Autodesk Fusion 360 part; units mm, degrees
note: some values were not read from the file. Set by a fixed rule: which sketch regions a step uses.
(part 6 of 59)
  spline S28 degree 5 poles (-28.1181, -0.5527) (-28.1154, -0.5525) (-28.11, -0.5521) (-28.1019, -0.5515) (-28.0911, -0.5506) (-28.0777, -0.5495) (-28.0644, -0.5484) (-28.051, -0.5473) (-28.0377, -0.5462) (-28.0244, -0.5451) (-28.0112, -0.5439) (-27.9979, -0.5427) (-27.9848, -0.5415) (-27.9716, -0.5404) (-27.9585, -0.5391) (-27.9454, -0.5379) (-27.9323, -0.5367) (-27.9193, -0.5354) (-27.9063, -0.5342) (-27.8934, -0.5329) (-27.8805, -0.5316) (-27.8676, -0.5303) (-27.8547, -0.529) (-27.8419, -0.5276) (-27.8291, -0.5263) (-27.8164, -0.5249) (-27.8037, -0.5236) (-27.791, -0.5222) (-27.7784, -0.5208) (-27.7658, -0.5194) (-27.7532, -0.518) (-27.7406, -0.5165) (-27.7281, -0.5151) (-27.7157, -0.5136) (-27.7032, -0.5122) (-27.6908, -0.5107) (-27.6785, -0.5092) (-27.6661, -0.5077) (-27.6539, -0.5062) (-27.6416, -0.5047) (-27.6294, -0.5031) (-27.6172, -0.5016) (-27.605, -0.5) (-27.5929, -0.4984) (-27.5809, -0.4968) (-27.5688, -0.4952) (-27.5568, -0.4936) (-27.5449, -0.492) (-27.5329, -0.4904) (-27.521, -0.4887) (-27.5092, -0.4871) (-27.4974, -0.4854) (-27.4856, -0.4838) (-27.4738, -0.4821) (-27.4621, -0.4804) (-27.4505, -0.4787) (-27.4388, -0.477) (-27.4273, -0.4752) (-27.4157, -0.4735) (-27.4042, -0.4718) (-27.3927, -0.47) (-27.3813, -0.4682) (-27.3699, -0.4665) (-27.3585, -0.4647) (-27.3472, -0.4629) (-27.3359, -0.4611) (-27.3247, -0.4593) (-27.3135, -0.4574) (-27.3023, -0.4556) (-27.2912, -0.4538) (-27.2801, -0.4519) (-27.2691, -0.4501) (-27.2581, -0.4482) (-27.2471, -0.4463) (-27.2362, -0.4445) (-27.2253, -0.4426) (-27.2145, -0.4407) (-27.2037, -0.4388) (-27.1929, -0.4368) (-27.1822, -0.4349) (-27.1715, -0.433) (-27.1609, -0.4311) (-27.1503, -0.4291) (-27.1397, -0.4272) (-27.1292, -0.4252) (-27.1188, -0.4232) (-27.1083, -0.4213) (-27.0979, -0.4193) (-27.0876, -0.4173) (-27.0773, -0.4153) (-27.0671, -0.4133) (-27.0568, -0.4113) (-27.0467, -0.4093) (-27.0365, -0.4072) (-27.0265, -0.4052) (-27.0164, -0.4032) (-27.0064, -0.4011) (-26.9965, -0.3991) (-26.9866, -0.3971) (-26.9767, -0.395) (-26.9669, -0.3929) (-26.9571, -0.3909) (-26.9474, -0.3888) (-26.9377, -0.3867) (-26.9281, -0.3847) (-26.9185, -0.3826) (-26.9089, -0.3805) (-26.8994, -0.3784) (-26.89, -0.3763) (-26.8806, -0.3742) (-26.8712, -0.3721) (-26.8619, -0.37) (-26.8526, -0.3679) (-26.8434, -0.3658) (-26.8342, -0.3636) (-26.8251, -0.3615) (-26.816, -0.3594) (-26.8069, -0.3573) (-26.798, -0.3551) (-26.789, -0.353) (-26.7801, -0.3509) (-26.7713, -0.3487) (-26.7625, -0.3466) (-26.7537, -0.3445) (-26.7451, -0.3423) (-26.7364, -0.3402) (-26.7278, -0.338) (-26.7193, -0.3359) (-26.7108, -0.3337) (-26.7023, -0.3316) (-26.6939, -0.3294) (-26.6856, -0.3273) (-26.6773, -0.3251) (-26.669, -0.323) (-26.6608, -0.3208) (-26.6527, -0.3187) (-26.6446, -0.3166) (-26.6365, -0.3144) (-26.6286, -0.3123) (-26.6206, -0.3101) (-26.6127, -0.308) (-26.6049, -0.3058) (-26.5971, -0.3037) (-26.5894, -0.3016) (-26.5817, -0.2994) (-26.5741, -0.2973) (-26.5665, -0.2952) (-26.559, -0.293) (-26.5516, -0.2909) (-26.5442, -0.2888) (-26.5368, -0.2867) (-26.5296, -0.2845) (-26.5223, -0.2824) (-26.5151, -0.2803) (-26.508, -0.2782) (-26.5009, -0.2761) (-26.4939, -0.274) (-26.487, -0.272) (-26.4801, -0.2699) (-26.4733, -0.2678) (-26.4665, -0.2657) (-26.4598, -0.2637) (-26.4531, -0.2616) (-26.4465, -0.2596) (-26.4399, -0.2575) (-26.4335, -0.2555) (-26.427, -0.2534) (-26.4207, -0.2514) (-26.4144, -0.2494) (-26.4081, -0.2474) (-26.4019, -0.2454) (-26.3958, -0.2434) (-26.3897, -0.2414) (-26.3837, -0.2395) (-26.3778, -0.2375) (-26.3719, -0.2356) (-26.3661, -0.2336) (-26.3604, -0.2317) (-26.3547, -0.2298) (-26.3491, -0.2279) (-26.3435, -0.226) (-26.338, -0.2241) (-26.3326, -0.2222) (-26.3273, -0.2204) (-26.322, -0.2185) (-26.3167, -0.2167) (-26.3116, -0.2149) (-26.3065, -0.2131) (-26.3015, -0.2113) (-26.2965, -0.2095) (-26.2916, -0.2077) (-26.2868, -0.206) (-26.282, -0.2043) (-26.2774, -0.2026) (-26.2728, -0.2009) (-26.2682, -0.1992) (-26.2638, -0.1975) (-26.2594, -0.1959) (-26.255, -0.1943) (-26.2508, -0.1927) (-26.2466, -0.1911) (-26.2425, -0.1895) (-26.2385, -0.188) (-26.2345, -0.1864) (-26.2307, -0.1849) (-26.2269, -0.1834) (-26.2231, -0.182) (-26.2195, -0.1806) (-26.2159, -0.1791) (-26.2124, -0.1778) (-26.209, -0.1764) (-26.2057, -0.175) (-26.2024, -0.1737) (-26.1993, -0.1724) (-26.1962, -0.1712) (-26.1932, -0.1699) (-26.1903, -0.1687) (-26.1874, -0.1676) (-26.1847, -0.1664) (-26.182, -0.1653) (-26.1794, -0.1642) (-26.1769, -0.1631) (-26.1745, -0.1621) (-26.1722, -0.1611) (-26.17, -0.1602) (-26.1678, -0.1592) (-26.1658, -0.1583) (-26.1638, -0.1575) (-26.1619, -0.1567) (-26.1602, -0.1559) (-26.1585, -0.1551) (-26.1569, -0.1544) (-26.1554, -0.1538) (-26.154, -0.1531) (-26.1527, -0.1526) (-26.1515, -0.152) (-26.1504, -0.1515) (-26.1495, -0.151) (-26.1486, -0.1506) (-26.1478, -0.1503) (-26.1471, -0.15) (-26.1467, -0.1497) (-26.1464, -0.1496) (-26.1462, -0.1495) (-26.1461, -0.1495) knots -1 -1 -1 -1 -1 -1 -0.99583333 -0.99166667 -0.9875 -0.98333333 -0.97916667 -0.975 -0.97083333 -0.96666667 -0.9625 -0.95833333 -0.95416667 -0.95 -0.94583333 -0.94166667 -0.9375 -0.93333333 -0.92916667 -0.925 -0.92083333 -0.91666667 -0.9125 -0.90833333 -0.90416667 -0.9 -0.89583333 -0.89166667 -0.8875 -0.88333333 -0.87916667 -0.875 -0.87083333 -0.86666667 -0.8625 -0.85833333 -0.85416667 -0.85 -0.84583333 -0.84166667 -0.8375 -0.83333333 -0.82916667 -0.825 -0.82083333 -0.81666667 -0.8125 -0.80833333 -0.80416667 -0.8 -0.79583333 -0.79166667 -0.7875 -0.78333333 -0.77916667 -0.775 -0.77083333 -0.76666667 -0.7625 -0.75833333 -0.75416667 -0.75 -0.74583333 -0.74166667 -0.7375 -0.73333333 -0.72916667 -0.725 -0.72083333 -0.71666667 -0.7125 -0.70833333 -0.70416667 -0.7 -0.69583333 -0.69166667 -0.6875 -0.68333333 -0.67916667 -0.675 -0.67083333 -0.66666667 -0.6625 -0.65833333 -0.65416667 -0.65 -0.64583333 -0.64166667 -0.6375 -0.63333333 -0.62916667 -0.625 -0.62083333 -0.61666667 -0.6125 -0.60833333 -0.60416667 -0.6 -0.59583333 -0.59166667 -0.5875 -0.58333333 -0.57916667 -0.575 -0.57083333 -0.56666667 -0.5625 -0.55833333 -0.55416667 -0.55 -0.54583333 -0.54166667 -0.5375 -0.53333333 -0.52916667 -0.525 -0.52083333 -0.51666667 -0.5125 -0.50833333 -0.50416667 -0.5 -0.49583333 -0.49166667 -0.4875 -0.48333333 -0.47916667 -0.475 -0.47083333 -0.46666667 -0.4625 -0.45833333 -0.45416667 -0.45 -0.44583333 -0.44166667 -0.4375 -0.43333333 -0.42916667 -0.425 -0.42083333 -0.41666667 -0.4125 -0.40833333 -0.40416667 -0.4 -0.39583333 -0.39166667 -0.3875 -0.38333333 -0.37916667 -0.375 -0.37083333 -0.36666667 -0.3625 -0.35833333 -0.35416667 -0.35 -0.34583333 -0.34166667 -0.3375 -0.33333333 -0.32916667 -0.325 -0.32083333 -0.31666667 -0.3125 -0.30833333 -0.30416667 -0.3 -0.29583333 -0.29166667 -0.2875 -0.28333333 -0.27916667 -0.275 -0.27083333 -0.26666667 -0.2625 -0.25833333 -0.25416667 -0.25 -0.24583333 -0.24166667 -0.2375 -0.23333333 -0.22916667 -0.225 -0.22083333 -0.21666667 -0.2125 -0.20833333 -0.20416667 -0.2 -0.19583333 -0.19166667 -0.1875 -0.18333333 -0.17916667 -0.175 -0.17083333 -0.16666667 -0.1625 -0.15833333 -0.15416667 -0.15 -0.14583333 -0.14166667 -0.1375 -0.13333333 -0.12916667 -0.125 -0.12083333 -0.11666667 -0.1125 -0.10833333 -0.10416667 -0.1 -0.09583333 -0.09166667 -0.0875 -0.08333333 -0.07916667 -0.075 -0.07083333 -0.06666667 -0.0625 -0.05833333 -0.05416667 -0.05 -0.04583333 -0.04166667 -0.0375 -0.03333333 -0.02916667 -0.025 -0.02083333 -0.01666667 -0.0125 -0.00833333 -0.00416667 0 0 0 0 0 0
  spline S29 degree 5 poles (-27.3251, 22.3472) (-27.3252, 22.3472) (-27.3254, 22.3473) (-27.3257, 22.3474) (-27.3262, 22.3475) (-27.3269, 22.3478) (-27.3277, 22.3481) (-27.3286, 22.3484) (-27.3296, 22.3487) (-27.3308, 22.3491) (-27.332, 22.3495) (-27.3334, 22.35) (-27.3348, 22.3505) (-27.3364, 22.351) (-27.338, 22.3515) (-27.3398, 22.3521) (-27.3416, 22.3527) (-27.3435, 22.3533) (-27.3456, 22.3539) (-27.3477, 22.3546) (-27.3499, 22.3553) (-27.3523, 22.356) (-27.3547, 22.3568) (-27.3572, 22.3575) (-27.3598, 22.3583) (-27.3625, 22.3591) (-27.3652, 22.36) (-27.3681, 22.3608) (-27.371, 22.3617) (-27.3741, 22.3626) (-27.3772, 22.3635) (-27.3804, 22.3645) (-27.3837, 22.3654) (-27.387, 22.3664) (-27.3905, 22.3674) (-27.394, 22.3684) (-27.3976, 22.3694) (-27.4013, 22.3704) (-27.4051, 22.3715) (-27.409, 22.3725) (-27.4129, 22.3736) (-27.4169, 22.3747) (-27.421, 22.3758) (-27.4252, 22.3769) (-27.4294, 22.378) (-27.4337, 22.3792) (-27.4381, 22.3803) (-27.4426, 22.3815) (-27.4471, 22.3827) (-27.4517, 22.3838) (-27.4564, 22.385) (-27.4612, 22.3862) (-27.466, 22.3874) (-27.4709, 22.3887) (-27.4759, 22.3899) (-27.481, 22.3911) (-27.4861, 22.3924) (-27.4912, 22.3936) (-27.4965, 22.3949) (-27.5018, 22.3962) (-27.5072, 22.3974) (-27.5127, 22.3987) (-27.5182, 22.4) (-27.5238, 22.4013) (-27.5294, 22.4026) (-27.5352, 22.4039) (-27.5409, 22.4052) (-27.5468, 22.4065) (-27.5527, 22.4079) (-27.5587, 22.4092) (-27.5647, 22.4105) (-27.5709, 22.4118) (-27.577, 22.4132) (-27.5833, 22.4145) (-27.5896, 22.4158) (-27.5959, 22.4172) (-27.6023, 22.4185) (-27.6088, 22.4199) (-27.6154, 22.4212) (-27.622, 22.4225) (-27.6286, 22.4239) (-27.6353, 22.4252) (-27.6421, 22.4266) (-27.649, 22.4279) (-27.6559, 22.4293) (-27.6628, 22.4306) (-27.6698, 22.432) (-27.6769, 22.4333) (-27.6841, 22.4347) (-27.6912, 22.436) (-27.6985, 22.4374) (-27.7058, 22.4387) (-27.7132, 22.4401) (-27.7206, 22.4414) (-27.728, 22.4428) (-27.7356, 22.4441) (-27.7431, 22.4454) (-27.7508, 22.4468) (-27.7585, 22.4481) (-27.7662, 22.4494) (-27.774, 22.4508) (-27.7819, 22.4521) (-27.7898, 22.4534) (-27.7977, 22.4547) (-27.8057, 22.456) (-27.8138, 22.4573) (-27.8219, 22.4586) (-27.8301, 22.4599) (-27.8383, 22.4612) (-27.8466, 22.4625) (-27.8549, 22.4638) (-27.8633, 22.4651) (-27.8717, 22.4664) (-27.8802, 22.4676) (-27.8887, 22.4689) (-27.8973, 22.4701) (-27.9059, 22.4714) (-27.9146, 22.4726) (-27.9233, 22.4739) (-27.9321, 22.4751) (-27.9409, 22.4763) (-27.9498, 22.4776) (-27.9587, 22.4788) (-27.9677, 22.48) (-27.9767, 22.4812) (-27.9858, 22.4824) (-27.9949, 22.4836) (-28.004, 22.4847) (-28.0133, 22.4859) (-28.0225, 22.4871) (-28.0318, 22.4882) (-28.0412, 22.4894) (-28.0506, 22.4905) (-28.06, 22.4916) (-28.0695, 22.4928) (-28.079, 22.4939) (-28.0886, 22.495) (-28.0982, 22.4961) (-28.1079, 22.4972) (-28.1176, 22.4983) (-28.1274, 22.4993) (-28.1372, 22.5004) (-28.147, 22.5014) (-28.1569, 22.5025) (-28.1668, 22.5035) (-28.1768, 22.5045) (-28.1868, 22.5055) (-28.1969, 22.5065) (-28.207, 22.5075) (-28.2172, 22.5085) (-28.2274, 22.5095) (-28.2376, 22.5104) (-28.2479, 22.5114) (-28.2582, 22.5123) (-28.2686, 22.5133) (-28.279, 22.5142) (-28.2894, 22.5151) (-28.2999, 22.516) (-28.3105, 22.5169) (-28.321, 22.5177) (-28.3317, 22.5186) (-28.3423, 22.5195) (-28.353, 22.5203) (-28.3638, 22.5211) (-28.3745, 22.5219) (-28.3854, 22.5227) (-28.3962, 22.5235) (-28.4071, 22.5243) (-28.4181, 22.5251) (-28.429, 22.5258) (-28.44, 22.5266) (-28.4511, 22.5273) (-28.4622, 22.528) (-28.4733, 22.5287) (-28.4845, 22.5294) (-28.4957, 22.5301) (-28.507, 22.5308) (-28.5183, 22.5314) (-28.5296, 22.5321) (-28.541, 22.5327) (-28.5524, 22.5333) (-28.5638, 22.5339) (-28.5753, 22.5345) (-28.5868, 22.5351) (-28.5984, 22.5356) (-28.61, 22.5362) (-28.6216, 22.5367) (-28.6333, 22.5372) (-28.645, 22.5377) (-28.6567, 22.5382) (-28.6685, 22.5387) (-28.6803, 22.5392) (-28.6922, 22.5396) (-28.7041, 22.54) (-28.716, 22.5405) (-28.728, 22.5409) (-28.74, 22.5412) (-28.752, 22.5416) (-28.7641, 22.542) (-28.7762, 22.5423) (-28.7883, 22.5427) (-28.8005, 22.543) (-28.8127, 22.5433) (-28.8249, 22.5436) (-28.8372, 22.5438) (-28.8495, 22.5441) (-28.8619, 22.5443) (-28.8743, 22.5445) (-28.8867, 22.5448) (-28.8991, 22.5449) (-28.9116, 22.5451) (-28.9241, 22.5453) (-28.9367, 22.5454) (-28.9493, 22.5456) (-28.9619, 22.5457) (-28.9745, 22.5458) (-28.9872, 22.5458) (-29, 22.5459) (-29.0127, 22.546) (-29.0255, 22.546) (-29.0383, 22.546) (-29.0512, 22.546) (-29.0641, 22.546) (-29.077, 22.546) (-29.0899, 22.5459) (-29.1029, 22.5458) (-29.1159, 22.5458) (-29.129, 22.5457) (-29.142, 22.5455) (-29.1551, 22.5454) (-29.1683, 22.5453) (-29.1815, 22.5451) (-29.1947, 22.5449) (-29.2079, 22.5447) (-29.2212, 22.5445) (-29.2345, 22.5442) (-29.2478, 22.544) (-29.2612, 22.5437) (-29.2745, 22.5434) (-29.288, 22.5431) (-29.3014, 22.5428) (-29.3122, 22.5425) (-29.3203, 22.5423) (-29.3257, 22.5422) (-29.3284, 22.5421) knots 0 0 0 0 0 0 0.00416667 0.00833333 0.0125 0.01666667 0.02083333 0.025 0.02916667 0.03333333 0.0375 0.04166667 0.04583333 0.05 0.05416667 0.05833333 0.0625 0.06666667 0.07083333 0.075 0.07916667 0.08333333 0.0875 0.09166667 0.09583333 0.1 0.10416667 0.10833333 0.1125 0.11666667 0.12083333 0.125 0.12916667 0.13333333 0.1375 0.14166667 0.14583333 0.15 0.15416667 0.15833333 0.1625 0.16666667 0.17083333 0.175 0.17916667 0.18333333 0.1875 0.19166667 0.19583333 0.2 0.20416667 0.20833333 0.2125 0.21666667 0.22083333 0.225 0.22916667 0.23333333 0.2375 0.24166667 0.24583333 0.25 0.25416667 0.25833333 0.2625 0.26666667 0.27083333 0.275 0.27916667 0.28333333 0.2875 0.29166667 0.29583333 0.3 0.30416667 0.30833333 0.3125 0.31666667 0.32083333 0.325 0.32916667 0.33333333 0.3375 0.34166667 0.34583333 0.35 0.35416667 0.35833333 0.3625 0.36666667 0.37083333 0.375 0.37916667 0.38333333 0.3875 0.39166667 0.39583333 0.4 0.40416667 0.40833333 0.4125 0.41666667 0.42083333 0.425 0.42916667 0.43333333 0.4375 0.44166667 0.44583333 0.45 0.45416667 0.45833333 0.4625 0.46666667 0.47083333 0.475 0.47916667 0.48333333 0.4875 0.49166667 0.49583333 0.5 0.50416667 0.50833333 0.5125 0.51666667 0.52083333 0.525 0.52916667 0.53333333 0.5375 0.54166667 0.54583333 0.55 0.55416667 0.55833333 0.5625 0.56666667 0.57083333 0.575 0.57916667 0.58333333 0.5875 0.59166667 0.59583333 0.6 0.60416667 0.60833333 0.6125 0.61666667 0.62083333 0.625 0.62916667 0.63333333 0.6375 0.64166667 0.64583333 0.65 0.65416667 0.65833333 0.6625 0.66666667 0.67083333 0.675 0.67916667 0.68333333 0.6875 0.69166667 0.69583333 0.7 0.70416667 0.70833333 0.7125 0.71666667 0.72083333 0.725 0.72916667 0.73333333 0.7375 0.74166667 0.74583333 0.75 0.75416667 0.75833333 0.7625 0.76666667 0.77083333 0.775 0.77916667 0.78333333 0.7875 0.79166667 0.79583333 0.8 0.80416667 0.80833333 0.8125 0.81666667 0.82083333 0.825 0.82916667 0.83333333 0.8375 0.84166667 0.84583333 0.85 0.85416667 0.85833333 0.8625 0.86666667 0.87083333 0.875 0.87916667 0.88333333 0.8875 0.89166667 0.89583333 0.9 0.90416667 0.90833333 0.9125 0.91666667 0.92083333 0.925 0.92916667 0.93333333 0.9375 0.94166667 0.94583333 0.95 0.95416667 0.95833333 0.9625 0.96666667 0.97083333 0.975 0.97916667 0.98333333 0.9875 0.99166667 0.99583333 1 1 1 1 1 1
  spline S30 degree 5 poles (-25.6019, -1.2175) (-25.602, -1.2175) (-25.6022, -1.2176) (-25.6025, -1.2178) (-25.6029, -1.218) (-25.6036, -1.2184) (-25.6043, -1.2188) (-25.6052, -1.2193) (-25.6061, -1.2198) (-25.6072, -1.2204) (-25.6083, -1.221) (-25.6096, -1.2217) (-25.6109, -1.2225) (-25.6123, -1.2233) (-25.6138, -1.2242) (-25.6154, -1.2251) (-25.6171, -1.2261) (-25.6188, -1.2271) (-25.6207, -1.2282) (-25.6226, -1.2293) (-25.6246, -1.2305) (-25.6267, -1.2317) (-25.6289, -1.233) (-25.6311, -1.2344) (-25.6334, -1.2358) (-25.6358, -1.2372) (-25.6383, -1.2387) (-25.6409, -1.2403) (-25.6435, -1.2419) (-25.6462, -1.2435) (-25.6489, -1.2452) (-25.6518, -1.247) (-25.6547, -1.2488) (-25.6577, -1.2506) (-25.6607, -1.2526) (-25.6638, -1.2545) (-25.667, -1.2565) (-25.6702, -1.2586) (-25.6735, -1.2607) (-25.6769, -1.2628) (-25.6803, -1.265) (-25.6838, -1.2673) (-25.6874, -1.2696) (-25.691, -1.2719) (-25.6947, -1.2743) (-25.6984, -1.2768) (-25.7022, -1.2793) (-25.706, -1.2818) (-25.71, -1.2844) (-25.7139, -1.287) (-25.718, -1.2897) (-25.722, -1.2925) (-25.7262, -1.2952) (-25.7304, -1.2981) (-25.7346, -1.3009) (-25.7389, -1.3039) (-25.7432, -1.3068) (-25.7476, -1.3098) (-25.7521, -1.3129) (-25.7566, -1.316) (-25.7612, -1.3192) (-25.7658, -1.3224) (-25.7704, -1.3256) (-25.7751, -1.3289) (-25.7799, -1.3322) (-25.7847, -1.3356) (-25.7895, -1.339) (-25.7944, -1.3425) (-25.7993, -1.346) (-25.8043, -1.3496) (-25.8093, -1.3532) (-25.8144, -1.3568) (-25.8195, -1.3605) (-25.8247, -1.3643) (-25.8299, -1.3681) (-25.8352, -1.3719) (-25.8405, -1.3758) (-25.8458, -1.3797) (-25.8512, -1.3836) (-25.8566, -1.3876) (-25.8621, -1.3917) (-25.8676, -1.3958) (-25.8731, -1.3999) (-25.8787, -1.4041) (-25.8843, -1.4083) (-25.89, -1.4126) (-25.8957, -1.4169) (-25.9014, -1.4213) (-25.9072, -1.4257) (-25.913, -1.4301) (-25.9188, -1.4346) (-25.9247, -1.4391) (-25.9306, -1.4437) (-25.9366, -1.4483) (-25.9426, -1.4529) (-25.9486, -1.4576) (-25.9547, -1.4624) (-25.9608, -1.4672) (-25.9669, -1.472) (-25.9731, -1.4769) (-25.9793, -1.4818) (-25.9855, -1.4867) (-25.9918, -1.4917) (-25.9981, -1.4967) (-26.0044, -1.5018) (-26.0108, -1.5069) (-26.0172, -1.5121) (-26.0236, -1.5173) (-26.0301, -1.5225) (-26.0366, -1.5278) (-26.0431, -1.5332) (-26.0497, -1.5385) (-26.0563, -1.5439) (-26.0629, -1.5494) (-26.0695, -1.5549) (-26.0762, -1.5604) (-26.0829, -1.566) (-26.0896, -1.5716) (-26.0964, -1.5772) (-26.1032, -1.5829) (-26.11, -1.5887) (-26.1168, -1.5945) (-26.1237, -1.6003) (-26.1306, -1.6061) (-26.1375, -1.612) (-26.1445, -1.618) (-26.1515, -1.6239) (-26.1585, -1.63) (-26.1655, -1.636) (-26.1726, -1.6421) (-26.1796, -1.6483) (-26.1868, -1.6544) (-26.1939, -1.6607) (-26.201, -1.6669) (-26.2082, -1.6732) (-26.2154, -1.6796) (-26.2227, -1.6859) (-26.2299, -1.6924) (-26.2372, -1.6988) (-26.2445, -1.7053) (-26.2518, -1.7119) (-26.2592, -1.7184) (-26.2665, -1.725) (-26.2739, -1.7317) (-26.2813, -1.7384) (-26.2888, -1.7451) (-26.2962, -1.7519) (-26.3037, -1.7587) (-26.3112, -1.7656) (-26.3188, -1.7724) (-26.3263, -1.7794) (-26.3339, -1.7863) (-26.3414, -1.7933) (-26.3491, -1.8004) (-26.3567, -1.8075) (-26.3643, -1.8146) (-26.372, -1.8217) (-26.3797, -1.8289) (-26.3874, -1.8362) (-26.3951, -1.8435) (-26.4029, -1.8508) (-26.4106, -1.8581) (-26.4184, -1.8655) (-26.4262, -1.8729) (-26.434, -1.8804) (-26.4419, -1.8879) (-26.4497, -1.8954) (-26.4576, -1.903) (-26.4655, -1.9106) (-26.4734, -1.9183) (-26.4813, -1.926) (-26.4893, -1.9337) (-26.4972, -1.9415) (-26.5052, -1.9493) (-26.5132, -1.9571) (-26.5212, -1.965) (-26.5292, -1.9729) (-26.5373, -1.9809) (-26.5453, -1.9889) (-26.5534, -1.9969) (-26.5615, -2.005) (-26.5696, -2.0131) (-26.5777, -2.0212) (-26.5858, -2.0294) (-26.594, -2.0376) (-26.6022, -2.0459) (-26.6103, -2.0541) (-26.6185, -2.0625) (-26.6267, -2.0708) (-26.635, -2.0792) (-26.6432, -2.0877) (-26.6514, -2.0961) (-26.6597, -2.1046) (-26.668, -2.1132) (-26.6763, -2.1218) (-26.6846, -2.1304) (-26.6929, -2.139) (-26.7012, -2.1477) (-26.7096, -2.1565) (-26.7179, -2.1652) (-26.7263, -2.174) (-26.7347, -2.1829) (-26.7431, -2.1917) (-26.7515, -2.2006) (-26.7599, -2.2096) (-26.7683, -2.2186) (-26.7767, -2.2276) (-26.7852, -2.2366) (-26.7937, -2.2457) (-26.8021, -2.2549) (-26.8106, -2.264) (-26.8191, -2.2732) (-26.8276, -2.2824) (-26.8361, -2.2917) (-26.8447, -2.301) (-26.8532, -2.3104) (-26.8618, -2.3197) (-26.8703, -2.3291) (-26.8789, -2.3386) (-26.8875, -2.3481) (-26.8961, -2.3576) (-26.9047, -2.3671) (-26.9133, -2.3767) (-26.9219, -2.3863) (-26.9305, -2.396) (-26.9392, -2.4057) (-26.9478, -2.4154) (-26.9565, -2.4252) (-26.9651, -2.435) (-26.9738, -2.4448) (-26.9825, -2.4547) (-26.9912, -2.4646) (-26.9999, -2.4745) (-27.0086, -2.4845) (-27.0173, -2.4945) (-27.026, -2.5045) (-27.0347, -2.5146) (-27.0435, -2.5247) (-27.0522, -2.5349) (-27.061, -2.545) (-27.0697, -2.5553) (-27.0767, -2.5635) (-27.082, -2.5696) (-27.0855, -2.5737) (-27.0873, -2.5758) knots 0 0 0 0 0 0 0.00416667 0.00833333 0.0125 0.01666667 0.02083333 0.025 0.02916667 0.03333333 0.0375 0.04166667 0.04583333 0.05 0.05416667 0.05833333 0.0625 0.06666667 0.07083333 0.075 0.07916667 0.08333333 0.0875 0.09166667 0.09583333 0.1 0.10416667 0.10833333 0.1125 0.11666667 0.12083333 0.125 0.12916667 0.13333333 0.1375 0.14166667 0.14583333 0.15 0.15416667 0.15833333 0.1625 0.16666667 0.17083333 0.175 0.17916667 0.18333333 0.1875 0.19166667 0.19583333 0.2 0.20416667 0.20833333 0.2125 0.21666667 0.22083333 0.225 0.22916667 0.23333333 0.2375 0.24166667 0.24583333 0.25 0.25416667 0.25833333 0.2625 0.26666667 0.27083333 0.275 0.27916667 0.28333333 0.2875 0.29166667 0.29583333 0.3 0.30416667 0.30833333 0.3125 0.31666667 0.32083333 0.325 0.32916667 0.33333333 0.3375 0.34166667 0.34583333 0.35 0.35416667 0.35833333 0.3625 0.36666667 0.37083333 0.375 0.37916667 0.38333333 0.3875 0.39166667 0.39583333 0.4 0.40416667 0.40833333 0.4125 0.41666667 0.42083333 0.425 0.42916667 0.43333333 0.4375 0.44166667 0.44583333 0.45 0.45416667 0.45833333 0.4625 0.46666667 0.47083333 0.475 0.47916667 0.48333333 0.4875 0.49166667 0.49583333 0.5 0.50416667 0.50833333 0.5125 0.51666667 0.52083333 0.525 0.52916667 0.53333333 0.5375 0.54166667 0.54583333 0.55 0.55416667 0.55833333 0.5625 0.56666667 0.57083333 0.575 0.57916667 0.58333333 0.5875 0.59166667 0.59583333 0.6 0.60416667 0.60833333 0.6125 0.61666667 0.62083333 0.625 0.62916667 0.63333333 0.6375 0.64166667 0.64583333 0.65 0.65416667 0.65833333 0.6625 0.66666667 0.67083333 0.675 0.67916667 0.68333333 0.6875 0.69166667 0.69583333 0.7 0.70416667 0.70833333 0.7125 0.71666667 0.72083333 0.725 0.72916667 0.73333333 0.7375 0.74166667 0.74583333 0.75 0.75416667 0.75833333 0.7625 0.76666667 0.77083333 0.775 0.77916667 0.78333333 0.7875 0.79166667 0.79583333 0.8 0.80416667 0.80833333 0.8125 0.81666667 0.82083333 0.825 0.82916667 0.83333333 0.8375 0.84166667 0.84583333 0.85 0.85416667 0.85833333 0.8625 0.86666667 0.87083333 0.875 0.87916667 0.88333333 0.8875 0.89166667 0.89583333 0.9 0.90416667 0.90833333 0.9125 0.91666667 0.92083333 0.925 0.92916667 0.93333333 0.9375 0.94166667 0.94583333 0.95 0.95416667 0.95833333 0.9625 0.96666667 0.97083333 0.975 0.97916667 0.98333333 0.9875 0.99166667 0.99583333 1 1 1 1 1 1
  arc A40 (-28.1181, 25.5527) -> (-28.5147, 24.6618) centre (0, 12.5) ccw
  arc A41 (-29.3284, 22.5421) -> (-29.6298, 21.6146) centre (0, 12.5) ccw
  spline S31 degree 5 poles (-26.1461, 25.1495) (-26.1462, 25.1495) (-26.1464, 25.1496) (-26.1467, 25.1497) (-26.1471, 25.15) (-26.1478, 25.1503) (-26.1486, 25.1506) (-26.1495, 25.151) (-26.1504, 25.1515) (-26.1515, 25.152) (-26.1527, 25.1526) (-26.154, 25.1531) (-26.1554, 25.1538) (-26.1569, 25.1544) (-26.1585, 25.1551) (-26.1602, 25.1559) (-26.1619, 25.1567) (-26.1638, 25.1575) (-26.1658, 25.1583) (-26.1678, 25.1592) (-26.17, 25.1602) (-26.1722, 25.1611) (-26.1745, 25.1621) (-26.1769, 25.1631) (-26.1794, 25.1642) (-26.182, 25.1653) (-26.1847, 25.1664) (-26.1874, 25.1676) (-26.1903, 25.1687) (-26.1932, 25.1699) (-26.1962, 25.1712) (-26.1993, 25.1724) (-26.2024, 25.1737) (-26.2057, 25.175) (-26.209, 25.1764) (-26.2124, 25.1778) (-26.2159, 25.1791) (-26.2195, 25.1806) (-26.2231, 25.182) (-26.2269, 25.1834) (-26.2307, 25.1849) (-26.2345, 25.1864) (-26.2385, 25.188) (-26.2425, 25.1895) (-26.2466, 25.1911) (-26.2508, 25.1927) (-26.255, 25.1943) (-26.2594, 25.1959) (-26.2638, 25.1975) (-26.2682, 25.1992) (-26.2728, 25.2009) (-26.2774, 25.2026) (-26.282, 25.2043) (-26.2868, 25.206) (-26.2916, 25.2077) (-26.2965, 25.2095) (-26.3015, 25.2113) (-26.3065, 25.2131) (-26.3116, 25.2149) (-26.3167, 25.2167) (-26.322, 25.2185) (-26.3273, 25.2204) (-26.3326, 25.2222) (-26.338, 25.2241) (-26.3435, 25.226) (-26.3491, 25.2279) (-26.3547, 25.2298) (-26.3604, 25.2317) (-26.3661, 25.2336) (-26.3719, 25.2356) (-26.3778, 25.2375) (-26.3837, 25.2395) (-26.3897, 25.2414) (-26.3958, 25.2434) (-26.4019, 25.2454) (-26.4081, 25.2474) (-26.4144, 25.2494) (-26.4207, 25.2514) (-26.427, 25.2534) (-26.4335, 25.2555) (-26.4399, 25.2575) (-26.4465, 25.2596) (-26.4531, 25.2616) (-26.4598, 25.2637) (-26.4665, 25.2657) (-26.4733, 25.2678) (-26.4801, 25.2699) (-26.487, 25.272) (-26.4939, 25.274) (-26.5009, 25.2761) (-26.508, 25.2782) (-26.5151, 25.2803) (-26.5223, 25.2824) (-26.5296, 25.2845) (-26.5368, 25.2867) (-26.5442, 25.2888) (-26.5516, 25.2909) (-26.559, 25.293) (-26.5665, 25.2952) (-26.5741, 25.2973) (-26.5817, 25.2994) (-26.5894, 25.3016) (-26.5971, 25.3037) (-26.6049, 25.3058) (-26.6127, 25.308) (-26.6206, 25.3101) (-26.6286, 25.3123) (-26.6365, 25.3144) (-26.6446, 25.3166) (-26.6527, 25.3187) (-26.6608, 25.3208) (-26.669, 25.323) (-26.6773, 25.3251) (-26.6856, 25.3273) (-26.6939, 25.3294) (-26.7023, 25.3316) (-26.7108, 25.3337) (-26.7193, 25.3359) (-26.7278, 25.338) (-26.7364, 25.3402) (-26.7451, 25.3423) (-26.7537, 25.3445) (-26.7625, 25.3466) (-26.7713, 25.3487) (-26.7801, 25.3509) (-26.789, 25.353) (-26.798, 25.3551) (-26.8069, 25.3573) (-26.816, 25.3594) (-26.8251, 25.3615) (-26.8342, 25.3636) (-26.8434, 25.3658) (-26.8526, 25.3679) (-26.8619, 25.37) (-26.8712, 25.3721) (-26.8806, 25.3742) (-26.89, 25.3763) (-26.8994, 25.3784) (-26.9089, 25.3805) (-26.9185, 25.3826) (-26.9281, 25.3847) (-26.9377, 25.3867) (-26.9474, 25.3888) (-26.9571, 25.3909) (-26.9669, 25.3929) (-26.9767, 25.395) (-26.9866, 25.3971) (-26.9965, 25.3991) (-27.0064, 25.4011) (-27.0164, 25.4032) (-27.0265, 25.4052) (-27.0365, 25.4072) (-27.0467, 25.4093) (-27.0568, 25.4113) (-27.0671, 25.4133) (-27.0773, 25.4153) (-27.0876, 25.4173) (-27.0979, 25.4193) (-27.1083, 25.4213) (-27.1188, 25.4232) (-27.1292, 25.4252) (-27.1397, 25.4272) (-27.1503, 25.4291) (-27.1609, 25.4311) (-27.1715, 25.433) (-27.1822, 25.4349) (-27.1929, 25.4368) (-27.2037, 25.4388) (-27.2145, 25.4407) (-27.2253, 25.4426) (-27.2362, 25.4445) (-27.2471, 25.4463) (-27.2581, 25.4482) (-27.2691, 25.4501) (-27.2801, 25.4519) (-27.2912, 25.4538) (-27.3023, 25.4556) (-27.3135, 25.4574) (-27.3247, 25.4593) (-27.3359, 25.4611) (-27.3472, 25.4629) (-27.3585, 25.4647) (-27.3699, 25.4665) (-27.3813, 25.4682) (-27.3927, 25.47) (-27.4042, 25.4718) (-27.4157, 25.4735) (-27.4273, 25.4752) (-27.4388, 25.477) (-27.4505, 25.4787) (-27.4621, 25.4804) (-27.4738, 25.4821) (-27.4856, 25.4838) (-27.4974, 25.4854) (-27.5092, 25.4871) (-27.521, 25.4887) (-27.5329, 25.4904) (-27.5449, 25.492) (-27.5568, 25.4936) (-27.5688, 25.4952) (-27.5809, 25.4968) (-27.5929, 25.4984) (-27.605, 25.5) (-27.6172, 25.5016) (-27.6294, 25.5031) (-27.6416, 25.5047) (-27.6539, 25.5062) (-27.6661, 25.5077) (-27.6785, 25.5092) (-27.6908, 25.5107) (-27.7032, 25.5122) (-27.7157, 25.5136) (-27.7281, 25.5151) (-27.7406, 25.5165) (-27.7532, 25.518) (-27.7658, 25.5194) (-27.7784, 25.5208) (-27.791, 25.5222) (-27.8037, 25.5236) (-27.8164, 25.5249) (-27.8291, 25.5263) (-27.8419, 25.5276) (-27.8547, 25.529) (-27.8676, 25.5303) (-27.8805, 25.5316) (-27.8934, 25.5329) (-27.9063, 25.5342) (-27.9193, 25.5354) (-27.9323, 25.5367) (-27.9454, 25.5379) (-27.9585, 25.5391) (-27.9716, 25.5404) (-27.9848, 25.5415) (-27.9979, 25.5427) (-28.0112, 25.5439) (-28.0244, 25.5451) (-28.0377, 25.5462) (-28.051, 25.5473) (-28.0644, 25.5484) (-28.0777, 25.5495) (-28.0911, 25.5506) (-28.1019, 25.5515) (-28.11, 25.5521) (-28.1154, 25.5525) (-28.1181, 25.5527) knots 0 0 0 0 0 0 0.00416667 0.00833333 0.0125 0.01666667 0.02083333 0.025 0.02916667 0.03333333 0.0375 0.04166667 0.04583333 0.05 0.05416667 0.05833333 0.0625 0.06666667 0.07083333 0.075 0.07916667 0.08333333 0.0875 0.09166667 0.09583333 0.1 0.10416667 0.10833333 0.1125 0.11666667 0.12083333 0.125 0.12916667 0.13333333 0.1375 0.14166667 0.14583333 0.15 0.15416667 0.15833333 0.1625 0.16666667 0.17083333 0.175 0.17916667 0.18333333 0.1875 0.19166667 0.19583333 0.2 0.20416667 0.20833333 0.2125 0.21666667 0.22083333 0.225 0.22916667 0.23333333 0.2375 0.24166667 0.24583333 0.25 0.25416667 0.25833333 0.2625 0.26666667 0.27083333 0.275 0.27916667 0.28333333 0.2875 0.29166667 0.29583333 0.3 0.30416667 0.30833333 0.3125 0.31666667 0.32083333 0.325 0.32916667 0.33333333 0.3375 0.34166667 0.34583333 0.35 0.35416667 0.35833333 0.3625 0.36666667 0.37083333 0.375 0.37916667 0.38333333 0.3875 0.39166667 0.39583333 0.4 0.40416667 0.40833333 0.4125 0.41666667 0.42083333 0.425 0.42916667 0.43333333 0.4375 0.44166667 0.44583333 0.45 0.45416667 0.45833333 0.4625 0.46666667 0.47083333 0.475 0.47916667 0.48333333 0.4875 0.49166667 0.49583333 0.5 0.50416667 0.50833333 0.5125 0.51666667 0.52083333 0.525 0.52916667 0.53333333 0.5375 0.54166667 0.54583333 0.55 0.55416667 0.55833333 0.5625 0.56666667 0.57083333 0.575 0.57916667 0.58333333 0.5875 0.59166667 0.59583333 0.6 0.60416667 0.60833333 0.6125 0.61666667 0.62083333 0.625 0.62916667 0.63333333 0.6375 0.64166667 0.64583333 0.65 0.65416667 0.65833333 0.6625 0.66666667 0.67083333 0.675 0.67916667 0.68333333 0.6875 0.69166667 0.69583333 0.7 0.70416667 0.70833333 0.7125 0.71666667 0.72083333 0.725 0.72916667 0.73333333 0.7375 0.74166667 0.74583333 0.75 0.75416667 0.75833333 0.7625 0.76666667 0.77083333 0.775 0.77916667 0.78333333 0.7875 0.79166667 0.79583333 0.8 0.80416667 0.80833333 0.8125 0.81666667 0.82083333 0.825 0.82916667 0.83333333 0.8375 0.84166667 0.84583333 0.85 0.85416667 0.85833333 0.8625 0.86666667 0.87083333 0.875 0.87916667 0.88333333 0.8875 0.89166667 0.89583333 0.9 0.90416667 0.90833333 0.9125 0.91666667 0.92083333 0.925 0.92916667 0.93333333 0.9375 0.94166667 0.94583333 0.95 0.95416667 0.95833333 0.9625 0.96666667 0.97083333 0.975 0.97916667 0.98333333 0.9875 0.99166667 0.99583333 1 1 1 1 1 1
  arc A42 (-20.7445, -7.4055) -> (-19.9055, -8.2445) centre (0, 12.5) ccw
  line L96 (-27.3243, 22.3469) -> (-27.3251, 22.3472)
  line L97 (-27.0473, 22.2471) -> (-27.3243, 22.3469)
  spline S32 degree 5 poles (-24.7898, -6.1136) (-24.7872, -6.1128) (-24.782, -6.1113) (-24.7743, -6.109) (-24.7639, -6.1059) (-24.751, -6.1021) (-24.7382, -6.0982) (-24.7253, -6.0943) (-24.7125, -6.0905) (-24.6998, -6.0866) (-24.6871, -6.0827) (-24.6744, -6.0788) (-24.6617, -6.0749) (-24.6491, -6.071) (-24.6365, -6.0671) (-24.624, -6.0632) (-24.6115, -6.0593) (-24.599, -6.0553) (-24.5866, -6.0514) (-24.5742, -6.0475) (-24.5618, -6.0435) (-24.5495, -6.0395) (-24.5372, -6.0356) (-24.5249, -6.0316) (-24.5127, -6.0277) (-24.5005, -6.0237) (-24.4884, -6.0197) (-24.4762, -6.0157) (-24.4642, -6.0117) (-24.4521, -6.0077) (-24.4401, -6.0037) (-24.4281, -5.9997) (-24.4162, -5.9957) (-24.4043, -5.9917) (-24.3925, -5.9877) (-24.3806, -5.9836) (-24.3689, -5.9796) (-24.3571, -5.9756) (-24.3454, -5.9715) (-24.3337, -5.9675) (-24.3221, -5.9634) (-24.3105, -5.9594) (-24.299, -5.9553) (-24.2874, -5.9513) (-24.276, -5.9472) (-24.2645, -5.9431) (-24.2531, -5.9391) (-24.2417, -5.935) (-24.2304, -5.9309) (-24.2191, -5.9269) (-24.2079, -5.9228) (-24.1967, -5.9187) (-24.1855, -5.9146) (-24.1744, -5.9105) (-24.1633, -5.9064) (-24.1522, -5.9023) (-24.1412, -5.8982) (-24.1302, -5.8941) (-24.1193, -5.89) (-24.1084, -5.8859) (-24.0975, -5.8818) (-24.0867, -5.8777) (-24.0759, -5.8736) (-24.0652, -5.8695) (-24.0545, -5.8654) (-24.0438, -5.8613) (-24.0332, -5.8572) (-24.0226, -5.8531) (-24.0121, -5.849) (-24.0016, -5.8449) (-23.9911, -5.8408) (-23.9807, -5.8366) (-23.9703, -5.8325) (-23.96, -5.8284) (-23.9497, -5.8243) (-23.9395, -5.8202) (-23.9292, -5.8161) (-23.9191, -5.812) (-23.909, -5.8079) (-23.8989, -5.8038) (-23.8888, -5.7996) (-23.8788, -5.7955) (-23.8689, -5.7914) (-23.859, -5.7873) (-23.8491, -5.7832) (-23.8393, -5.7791) (-23.8295, -5.775) (-23.8197, -5.7709) (-23.81, -5.7668) (-23.8004, -5.7627) (-23.7907, -5.7587) (-23.7812, -5.7546) (-23.7716, -5.7505) (-23.7622, -5.7464) (-23.7527, -5.7423) (-23.7433, -5.7383) (-23.734, -5.7342) (-23.7247, -5.7301) (-23.7154, -5.726) (-23.7062, -5.722) (-23.697, -5.7179) (-23.6879, -5.7139) (-23.6788, -5.7098) (-23.6697, -5.7058) (-23.6607, -5.7018) (-23.6518, -5.6977) (-23.6429, -5.6937) (-23.634, -5.6897) (-23.6252, -5.6857) (-23.6165, -5.6816) (-23.6077, -5.6776) (-23.5991, -5.6736) (-23.5904, -5.6696) (-23.5818, -5.6657) (-23.5733, -5.6617) (-23.5648, -5.6577) (-23.5564, -5.6537) (-23.548, -5.6498) (-23.5396, -5.6458) (-23.5313, -5.6419) (-23.5231, -5.6379) (-23.5149, -5.634) (-23.5067, -5.6301) (-23.4986, -5.6262) (-23.4905, -5.6223) (-23.4825, -5.6184) (-23.4746, -5.6145) (-23.4666, -5.6106) (-23.4588, -5.6068) (-23.451, -5.6029) (-23.4432, -5.5991) (-23.4355, -5.5952) (-23.4278, -5.5914) (-23.4202, -5.5876) (-23.4126, -5.5838) (-23.4051, -5.58) (-23.3976, -5.5762) (-23.3902, -5.5724) (-23.3828, -5.5687) (-23.3755, -5.5649) (-23.3683, -5.5612) (-23.361, -5.5575) (-23.3539, -5.5538) (-23.3468, -5.5501) (-23.3397, -5.5464) (-23.3327, -5.5427) (-23.3257, -5.539) (-23.3188, -5.5354) (-23.312, -5.5318) (-23.3052, -5.5282) (-23.2984, -5.5246) (-23.2918, -5.521) (-23.2851, -5.5174) (-23.2785, -5.5139) (-23.272, -5.5103) (-23.2655, -5.5068) (-23.2591, -5.5033) (-23.2527, -5.4998) (-23.2464, -5.4963) (-23.2402, -5.4929) (-23.234, -5.4895) (-23.2278, -5.486) (-23.2217, -5.4826) (-23.2157, -5.4793) (-23.2097, -5.4759) (-23.2038, -5.4726) (-23.1979, -5.4692) (-23.1921, -5.4659) (-23.1864, -5.4627) (-23.1807, -5.4594) (-23.1751, -5.4562) (-23.1695, -5.4529) (-23.164, -5.4497) (-23.1585, -5.4466) (-23.1531, -5.4434) (-23.1478, -5.4403) (-23.1425, -5.4372) (-23.1373, -5.4341) (-23.1321, -5.431) (-23.127, -5.428) (-23.122, -5.425) (-23.117, -5.422) (-23.1121, -5.4191) (-23.1072, -5.4161) (-23.1024, -5.4132) (-23.0977, -5.4103) (-23.093, -5.4075) (-23.0884, -5.4047) (-23.0839, -5.4019) (-23.0794, -5.3991) (-23.075, -5.3964) (-23.0706, -5.3937) (-23.0664, -5.391) (-23.0621, -5.3883) (-23.058, -5.3857) (-23.0539, -5.3831) (-23.0499, -5.3806) (-23.0459, -5.3781) (-23.042, -5.3756) (-23.0382, -5.3731) (-23.0344, -5.3707) (-23.0308, -5.3683) (-23.0271, -5.366) (-23.0236, -5.3637) (-23.0201, -5.3614) (-23.0167, -5.3592) (-23.0134, -5.357) (-23.0101, -5.3548) (-23.0069, -5.3527) (-23.0038, -5.3506) (-23.0007, -5.3485) (-22.9978, -5.3465) (-22.9948, -5.3446) (-22.992, -5.3427) (-22.9893, -5.3408) (-22.9866, -5.3389) (-22.984, -5.3372) (-22.9814, -5.3354) (-22.979, -5.3337) (-22.9766, -5.3321) (-22.9743, -5.3305) (-22.9721, -5.3289) (-22.9699, -5.3274) (-22.9679, -5.326) (-22.9659, -5.3246) (-22.964, -5.3232) (-22.9622, -5.3219) (-22.9604, -5.3207) (-22.9588, -5.3195) (-22.9572, -5.3183) (-22.9557, -5.3172) (-22.9543, -5.3162) (-22.953, -5.3153) (-22.9518, -5.3144) (-22.9506, -5.3135) (-22.9496, -5.3127) (-22.9486, -5.312) (-22.9477, -5.3114) (-22.9469, -5.3108) (-22.9463, -5.3103) (-22.9457, -5.3098) (-22.9453, -5.3095) (-22.945, -5.3093) (-22.9448, -5.3092) (-22.9448, -5.3091) knots -1 -1 -1 -1 -1 -1 -0.99583333 -0.99166667 -0.9875 -0.98333333 -0.97916667 -0.975 -0.97083333 -0.96666667 -0.9625 -0.95833333 -0.95416667 -0.95 -0.94583333 -0.94166667 -0.9375 -0.93333333 -0.92916667 -0.925 -0.92083333 -0.91666667 -0.9125 -0.90833333 -0.90416667 -0.9 -0.89583333 -0.89166667 -0.8875 -0.88333333 -0.87916667 -0.875 -0.87083333 -0.86666667 -0.8625 -0.85833333 -0.85416667 -0.85 -0.84583333 -0.84166667 -0.8375 -0.83333333 -0.82916667 -0.825 -0.82083333 -0.81666667 -0.8125 -0.80833333 -0.80416667 -0.8 -0.79583333 -0.79166667 -0.7875 -0.78333333 -0.77916667 -0.775 -0.77083333 -0.76666667 -0.7625 -0.75833333 -0.75416667 -0.75 -0.74583333 -0.74166667 -0.7375 -0.73333333 -0.72916667 -0.725 -0.72083333 -0.71666667 -0.7125 -0.70833333 -0.70416667 -0.7 -0.69583333 -0.69166667 -0.6875 -0.68333333 -0.67916667 -0.675 -0.67083333 -0.66666667 -0.6625 -0.65833333 -0.65416667 -0.65 -0.64583333 -0.64166667 -0.6375 -0.63333333 -0.62916667 -0.625 -0.62083333 -0.61666667 -0.6125 -0.60833333 -0.60416667 -0.6 -0.59583333 -0.59166667 -0.5875 -0.58333333 -0.57916667 -0.575 -0.57083333 -0.56666667 -0.5625 -0.55833333 -0.55416667 -0.55 -0.54583333 -0.54166667 -0.5375 -0.53333333 -0.52916667 -0.525 -0.52083333 -0.51666667 -0.5125 -0.50833333 -0.50416667 -0.5 -0.49583333 -0.49166667 -0.4875 -0.48333333 -0.47916667 -0.475 -0.47083333 -0.46666667 -0.4625 -0.45833333 -0.45416667 -0.45 -0.44583333 -0.44166667 -0.4375 -0.43333333 -0.42916667 -0.425 -0.42083333 -0.41666667 -0.4125 -0.40833333 -0.40416667 -0.4 -0.39583333 -0.39166667 -0.3875 -0.38333333 -0.37916667 -0.375 -0.37083333 -0.36666667 -0.3625 -0.35833333 -0.35416667 -0.35 -0.34583333 -0.34166667 -0.3375 -0.33333333 -0.32916667 -0.325 -0.32083333 -0.31666667 -0.3125 -0.30833333 -0.30416667 -0.3 -0.29583333 -0.29166667 -0.2875 -0.28333333 -0.27916667 -0.275 -0.27083333 -0.26666667 -0.2625 -0.25833333 -0.25416667 -0.25 -0.24583333 -0.24166667 -0.2375 -0.23333333 -0.22916667 -0.225 -0.22083333 -0.21666667 -0.2125 -0.20833333 -0.20416667 -0.2 -0.19583333 -0.19166667 -0.1875 -0.18333333 -0.17916667 -0.175 -0.17083333 -0.16666667 -0.1625 -0.15833333 -0.15416667 -0.15 -0.14583333 -0.14166667 -0.1375 -0.13333333 -0.12916667 -0.125 -0.12083333 -0.11666667 -0.1125 -0.10833333 -0.10416667 -0.1 -0.09583333 -0.09166667 -0.0875 -0.08333333 -0.07916667 -0.075 -0.07083333 -0.06666667 -0.0625 -0.05833333 -0.05416667 -0.05 -0.04583333 -0.04166667 -0.0375 -0.03333333 -0.02916667 -0.025 -0.02083333 -0.01666667 -0.0125 -0.00833333 -0.00416667 0 0 0 0 0 0
  line L98 (-28.2972, 7.4176) -> (-28.587, 7.3655)
  arc A43 (-25.3417, 26.078) -> (-25.8803, 25.0209) centre (0, 12.5) ccw
  spline S33 degree 5 poles (-28.9679, 10.3817) (-28.968, 10.3817) (-28.9682, 10.3817) (-28.9685, 10.3817) (-28.969, 10.3816) (-28.9698, 10.3816) (-28.9706, 10.3815) (-28.9716, 10.3814) (-28.9727, 10.3813) (-28.9739, 10.3812) (-28.9752, 10.3811) (-28.9766, 10.3809) (-28.9781, 10.3808) (-28.9798, 10.3806) (-28.9815, 10.3804) (-28.9833, 10.3802) (-28.9852, 10.38) (-28.9873, 10.3798) (-28.9894, 10.3796) (-28.9916, 10.3793) (-28.9939, 10.379) (-28.9963, 10.3788) (-28.9989, 10.3785) (-29.0015, 10.3781) (-29.0041, 10.3778) (-29.0069, 10.3775) (-29.0098, 10.3771) (-29.0128, 10.3767) (-29.0158, 10.3763) (-29.0189, 10.3759) (-29.0222, 10.3755) (-29.0255, 10.375) (-29.0289, 10.3746) (-29.0323, 10.3741) (-29.0359, 10.3736) (-29.0395, 10.373) (-29.0432, 10.3725) (-29.047, 10.3719) (-29.0509, 10.3714) (-29.0549, 10.3708) (-29.0589, 10.3701) (-29.063, 10.3695) (-29.0672, 10.3688) (-29.0714, 10.3682) (-29.0758, 10.3675) (-29.0802, 10.3668) (-29.0847, 10.366) (-29.0892, 10.3653) (-29.0938, 10.3645) (-29.0985, 10.3637) (-29.1033, 10.3629) (-29.1081, 10.362) (-29.1131, 10.3612) (-29.118, 10.3603) (-29.1231, 10.3594) (-29.1282, 10.3585) (-29.1334, 10.3576) (-29.1386, 10.3566) (-29.1439, 10.3556) (-29.1493, 10.3546) (-29.1547, 10.3536) (-29.1602, 10.3525) (-29.1658, 10.3515) (-29.1714, 10.3504) (-29.1771, 10.3493) (-29.1829, 10.3481) (-29.1887, 10.347) (-29.1946, 10.3458) (-29.2005, 10.3446) (-29.2065, 10.3433) (-29.2126, 10.3421) (-29.2187, 10.3408) (-29.2249, 10.3395) (-29.2311, 10.3382) (-29.2374, 10.3369) (-29.2438, 10.3355) (-29.2502, 10.3341) (-29.2567, 10.3327) (-29.2632, 10.3313) (-29.2698, 10.3298) (-29.2764, 10.3284) (-29.2831, 10.3269) (-29.2899, 10.3253) (-29.2967, 10.3238) (-29.3035, 10.3222) (-29.3104, 10.3206) (-29.3174, 10.319) (-29.3244, 10.3173) (-29.3314, 10.3157) (-29.3386, 10.314) (-29.3457, 10.3123) (-29.3529, 10.3105) (-29.3602, 10.3088) (-29.3675, 10.307) (-29.3749, 10.3052) (-29.3823, 10.3033) (-29.3898, 10.3015) (-29.3973, 10.2996) (-29.4049, 10.2977) (-29.4125, 10.2957) (-29.4202, 10.2938) (-29.4279, 10.2918) (-29.4356, 10.2898) (-29.4434, 10.2877) (-29.4513, 10.2857) (-29.4592, 10.2836) (-29.4671, 10.2815) (-29.4751, 10.2793) (-29.4832, 10.2772) (-29.4912, 10.275) (-29.4994, 10.2728) (-29.5075, 10.2705) (-29.5158, 10.2683) (-29.524, 10.266) (-29.5323, 10.2637) (-29.5407, 10.2613) (-29.5491, 10.259) (-29.5575, 10.2566) (-29.566, 10.2542) (-29.5745, 10.2517) (-29.583, 10.2492) (-29.5917, 10.2467) (-29.6003, 10.2442) (-29.609, 10.2417) (-29.6177, 10.2391) (-29.6265, 10.2365) (-29.6353, 10.2339) (-29.6441, 10.2312) (-29.653, 10.2286) (-29.6619, 10.2259) (-29.6709, 10.2231) (-29.6799, 10.2204) (-29.689, 10.2176) (-29.6981, 10.2148) (-29.7072, 10.212) (-29.7163, 10.2091) (-29.7255, 10.2062) (-29.7348, 10.2033) (-29.7441, 10.2004) (-29.7534, 10.1974) (-29.7627, 10.1944) (-29.7721, 10.1914) (-29.7815, 10.1883) (-29.791, 10.1853) (-29.8005, 10.1822) (-29.81, 10.179) (-29.8196, 10.1759) (-29.8292, 10.1727) (-29.8388, 10.1695) (-29.8485, 10.1663) (-29.8582, 10.163) (-29.868, 10.1597) (-29.8777, 10.1564) (-29.8875, 10.1531) (-29.8974, 10.1497) (-29.9073, 10.1463) (-29.9172, 10.1429) (-29.9271, 10.1394) (-29.9371, 10.136) (-29.9471, 10.1325) (-29.9572, 10.1289) (-29.9673, 10.1254) (-29.9774, 10.1218) (-29.9875, 10.1182) (-29.9977, 10.1145) (-30.0079, 10.1109) (-30.0182, 10.1072) (-30.0284, 10.1035) (-30.0388, 10.0997) (-30.0491, 10.0959) (-30.0595, 10.0921) (-30.0699, 10.0883) (-30.0803, 10.0844) (-30.0907, 10.0806) (-30.1012, 10.0766) (-30.1118, 10.0727) (-30.1223, 10.0687) (-30.1329, 10.0647) (-30.1435, 10.0607) (-30.1541, 10.0567) (-30.1648, 10.0526) (-30.1755, 10.0485) (-30.1862, 10.0443) (-30.197, 10.0402) (-30.2078, 10.036) (-30.2186, 10.0318) (-30.2294, 10.0275) (-30.2403, 10.0233) (-30.2512, 10.019) (-30.2621, 10.0146) (-30.2731, 10.0103) (-30.2841, 10.0059) (-30.2951, 10.0015) (-30.3061, 9.997) (-30.3172, 9.9926) (-30.3283, 9.9881) (-30.3394, 9.9835) (-30.3506, 9.979) (-30.3617, 9.9744) (-30.3729, 9.9698) (-30.3841, 9.9652) (-30.3954, 9.9605) (-30.4067, 9.9558) (-30.418, 9.9511) (-30.4293, 9.9463) (-30.4407, 9.9416) (-30.452, 9.9368) (-30.4634, 9.9319) (-30.4749, 9.9271) (-30.4863, 9.9222) (-30.4978, 9.9173) (-30.5093, 9.9123) (-30.5208, 9.9073) (-30.5324, 9.9023) (-30.5439, 9.8973) (-30.5555, 9.8923) (-30.5672, 9.8872) (-30.5788, 9.8821) (-30.5905, 9.8769) (-30.6022, 9.8717) (-30.6139, 9.8665) (-30.6256, 9.8613) (-30.6374, 9.8561) (-30.6492, 9.8508) (-30.661, 9.8455) (-30.6728, 9.8401) (-30.6847, 9.8347) (-30.6966, 9.8293) (-30.7085, 9.8239) (-30.7204, 9.8185) (-30.7323, 9.813) (-30.7443, 9.8075) (-30.7563, 9.8019) (-30.7683, 9.7964) (-30.7803, 9.7908) (-30.7924, 9.7851) (-30.8044, 9.7795) (-30.8165, 9.7738) (-30.8287, 9.7681) (-30.8408, 9.7624) (-30.853, 9.7566) (-30.8627, 9.752) (-30.87, 9.7485) (-30.8749, 9.7461) (-30.8773, 9.745) knots 0 0 0 0 0 0 0.00416667 0.00833333 0.0125 0.01666667 0.02083333 0.025 0.02916667 0.03333333 0.0375 0.04166667 0.04583333 0.05 0.05416667 0.05833333 0.0625 0.06666667 0.07083333 0.075 0.07916667 0.08333333 0.0875 0.09166667 0.09583333 0.1 0.10416667 0.10833333 0.1125 0.11666667 0.12083333 0.125 0.12916667 0.13333333 0.1375 0.14166667 0.14583333 0.15 0.15416667 0.15833333 0.1625 0.16666667 0.17083333 0.175 0.17916667 0.18333333 0.1875 0.19166667 0.19583333 0.2 0.20416667 0.20833333 0.2125 0.21666667 0.22083333 0.225 0.22916667 0.23333333 0.2375 0.24166667 0.24583333 0.25 0.25416667 0.25833333 0.2625 0.26666667 0.27083333 0.275 0.27916667 0.28333333 0.2875 0.29166667 0.29583333 0.3 0.30416667 0.30833333 0.3125 0.31666667 0.32083333 0.325 0.32916667 0.33333333 0.3375 0.34166667 0.34583333 0.35 0.35416667 0.35833333 0.3625 0.36666667 0.37083333 0.375 0.37916667 0.38333333 0.3875 0.39166667 0.39583333 0.4 0.40416667 0.40833333 0.4125 0.41666667 0.42083333 0.425 0.42916667 0.43333333 0.4375 0.44166667 0.44583333 0.45 0.45416667 0.45833333 0.4625 0.46666667 0.47083333 0.475 0.47916667 0.48333333 0.4875 0.49166667 0.49583333 0.5 0.50416667 0.50833333 0.5125 0.51666667 0.52083333 0.525 0.52916667 0.53333333 0.5375 0.54166667 0.54583333 0.55 0.55416667 0.55833333 0.5625 0.56666667 0.57083333 0.575 0.57916667 0.58333333 0.5875 0.59166667 0.59583333 0.6 0.60416667 0.60833333 0.6125 0.61666667 0.62083333 0.625 0.62916667 0.63333333 0.6375 0.64166667 0.64583333 0.65 0.65416667 0.65833333 0.6625 0.66666667 0.67083333 0.675 0.67916667 0.68333333 0.6875 0.69166667 0.69583333 0.7 0.70416667 0.70833333 0.7125 0.71666667 0.72083333 0.725 0.72916667 0.73333333 0.7375 0.74166667 0.74583333 0.75 0.75416667 0.75833333 0.7625 0.76666667 0.77083333 0.775 0.77916667 0.78333333 0.7875 0.79166667 0.79583333 0.8 0.80416667 0.80833333 0.8125 0.81666667 0.82083333 0.825 0.82916667 0.83333333 0.8375 0.84166667 0.84583333 0.85 0.85416667 0.85833333 0.8625 0.86666667 0.87083333 0.875 0.87916667 0.88333333 0.8875 0.89166667 0.89583333 0.9 0.90416667 0.90833333 0.9125 0.91666667 0.92083333 0.925 0.92916667 0.93333333 0.9375 0.94166667 0.94583333 0.95 0.95416667 0.95833333 0.9625 0.96666667 0.97083333 0.975 0.97916667 0.98333333 0.9875 0.99166667 0.99583333 1 1 1 1 1 1
  arc A44 (-28.7355, 11.5881) -> (-28.6734, 10.4033) centre (0, 12.5) ccw